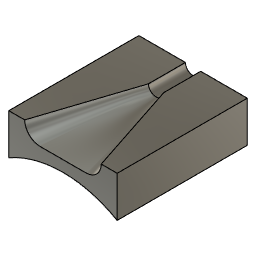
NCV-08 v2 (Autodesk Fusion 360 design; units mm, degrees)
Autodesk Fusion 360 part; units mm, degrees
sketch "Sketch1" plane through (0, 0, 0) normal (0, 1, 0) x (1, 0, 0)
  line L0 (-42.5, 0) -> (42.5, 0)
  line L1 (42.5, 0) -> (42.5, -32)
  line L2 (42.5, -32) -> (-42.5, -32)
  line L3 (-42.5, -32) -> (-42.5, 0)
  arc A0 (-42.5, 0) -> (42.5, 0) centre (0, 73.6122) ccw
  line L4 (-30, -32) -> (30, -32)
  line L5 (18, -20) -> (-18, -20)
  arc A1 (-18, -20) -> (-30, -32) centre (-18, -32) ccw
  arc A2 (30, -32) -> (18, -20) centre (18, -32) ccw
  arc A3 (6, -32) -> (-6, -32) centre (0, -32) ccw
  dimension "d1" = 42.5
  dimension "d2" = 42.5
  dimension "d3" = 32
  dimension "d4" = 32
  dimension "d5" = 170
  dimension "d6" = 20
  dimension "d9" = 12
  dimension "d10" = 12
  dimension "d11" = 30
  dimension "d12" = 30
  dimension "d13" = 12
  dimension "d14" = 42.5
  constraint horizontal L0
  constraint vertical L1
  constraint horizontal L2
  constraint vertical L3
  constraint horizontal L4
  constraint horizontal L5
  constraint coincident L2 L4.start
  constraint tangent L5 A1
  constraint coincident L4.start A1.end
  constraint tangent L5 A2
  constraint coincident L4.end A2.start
  constraint coincident L2 A3.centre
  constraint coincident L2 A3.end
  constraint coincident L2 A3.start
  measures "d1" distance of origin L3
  measures "d2" distance of origin L1
  measures "d3" distance of origin L2
  measures "d4" distance of L0 L2
  measures "d5" diameter of A0
  measures "d6" distance of origin L5
  measures "d9" radius of A1
  measures "d10" radius of A2
  measures "d11" horizontal distance of origin L4.start
  measures "d12" horizontal distance of origin L4.end
  measures "d13" diameter of A3
  measures "d14" distance of L1 A3.centre
extrude "Extrude1" add sketch "Sketch1" along normal blind 102 contours L1 L2 L3 A0 L5 A1 A2 | L2 L4 L5 A1 A2 A3
extrude "Extrude2" add sketch "Sketch1" along normal blind 73 contours L2 L4 A3
loft "Loft1" cut profiles "Sketch1" section 1 contours L2 L4 L5 A1 A2 A3 | L2 L4 A3 section 2 face at (-0.1495, 73, 30.0056)
equation "d1 = ( 85 / 2 ) * 1 mm"
equation "d2 = ( 85 / 2 ) * 1 mm"
equation "d5 = ( 85 * 2 ) * 1 mm"
equation "d14 = d2"
equation "d17 = 102 mm - 29 mm"
